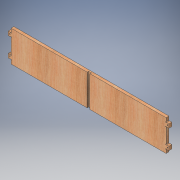
# Autodesk Inventor part: shelf
Saved by Autodesk Inventor 2016 (Build 200138000, 138)
## iProperties
Created: 2017-03-13
Part Number: shelf
Material: Wood (Birch)
Document SubType Name: Modeling
Designer: jwillauer
Density: 0.55 g/cm^3
Appearance: Birch - Natural Polished
Author: jwillauer
Autodesk Inventor part; units mm, degrees
ref_plane "YZ Plane" through (0, 0, 0) normal (1, 0, 0) x (0, 1, 0)
ref_plane "XZ Plane" through (0, 0, 0) normal (0, 1, 0) x (-1, 0, 0)
ref_plane "XY Plane" through (0, 0, 0) normal (0, 0, 1) x (1, 0, 0)
sketch "Sketch1" plane through (0, 0, 0) normal (0, 0, 1) x (1, 0, 0)
  line L0 (-759.3317, 185.2455) -> (256.6683, 185.2455)
  line L1 (-759.3317, -17.9545) -> (256.6683, -17.9545)
  line L2 (-759.3317, 185.2455) -> (-759.3317, 159.8455)
  line L3 (-759.3317, 159.8455) -> (-778.1277, 159.8455)
  line L4 (-778.1277, 159.8455) -> (-778.1277, 134.4455)
  line L5 (-778.1277, 134.4455) -> (-759.3317, 134.4455)
  line L6 (-759.3317, 134.4455) -> (-759.3317, 32.8455)
  line L7 (-759.3317, 32.8455) -> (-778.1277, 32.8455)
  line L8 (-778.1277, 32.8455) -> (-778.1277, 7.4455)
  line L9 (-778.1277, 7.4455) -> (-759.3317, 7.4455)
  line L10 (-759.3317, 7.4455) -> (-759.3317, -17.9545)
  line L11 (256.6683, 185.2455) -> (256.6683, 159.8455)
  line L12 (256.6683, 159.8455) -> (275.4643, 159.8455)
  line L13 (275.4643, 159.8455) -> (275.4643, 134.4455)
  line L14 (275.4643, 134.4455) -> (256.6683, 134.4455)
  line L15 (256.6683, 134.4455) -> (256.6683, 32.8455)
  line L16 (256.6683, 32.8455) -> (275.4643, 32.8455)
  line L17 (275.4643, 32.8455) -> (275.4643, 7.4455)
  line L18 (275.4643, 7.4455) -> (256.6683, 7.4455)
  line L19 (256.6683, 7.4455) -> (256.6683, -17.9545)
  point P0 (0, 0)
  dimension "d0" = 1016
  dimension "d1" = 203.2
  dimension "d2" = 25.4
  dimension "d3" = 25.4
  dimension "d4" = 25.4
  dimension "d5" = 25.4
  dimension "d6" = 18.796
  dimension "d7" = 18.796
  dimension "d8" = 18.796
  dimension "d9" = 25.4
  dimension "d11" = 25.4
  dimension "d12" = 25.4
  dimension "d15" = 25.4
  constraints: 40 end point, 12 perpendicular, 8 point on line, 2 parallel, 2 vertical, 1 horizontal
  measures "d0" distance of L0.start L0.end
  measures "d1" distance between parallel lines of L0 L1
  measures "d2" distance of L0.start L2.end
  measures "d3" distance of L3.end L4.end
  measures "d4" distance of L9.end L1.start
  measures "d5" distance of L7.end L8.end
  measures "d6" distance of L6.end L7.end
  measures "d7" distance of L8.end L9.end
  measures "d8" distance of L11.end L12.end
  measures "d9" distance of L0.end L11.end
  measures "d11" distance of L16.end L17.end
  measures "d12" distance of L12.end L13.end
  measures "d15" distance of L18.end L1.end
extrude "Extrusion1" add sketch "Sketch1" along normal blind 18.796
sketch "Sketch2" plane through (0, 0, 18.796) normal (0, 0, 1) x (1, 0, 0)
  line L0 (-778.1277, 159.8455) -> (-759.3317, 159.8455) projected
  line L1 (275.4643, 159.8455) -> (256.6683, 159.8455) projected
  point P0 (0, 0)
  point P1 (-759.3317, 134.5414)
  point P2 (-759.3317, 32.5902)
  point P3 (-759.3317, 7.3202)
  point P4 (256.6683, 134.5414)
  point P5 (256.6683, 32.5902)
  point P6 (256.6683, 7.3202)
hole "Hole1" at (-759.3317, 159.8455, 18.796) at (-759.3317, 134.5414, 18.796) at (-759.3317, 32.5902, 18.796) at (-759.3317, 7.3202, 18.796) at (256.6683, 159.8455, 18.796) at (256.6683, 134.5414, 18.796) at (256.6683, 32.5902, 18.796) at (256.6683, 7.3202, 18.796) direction (0, 0, -1) diameter 6.35 end through all
sketch "Sketch3" plane through (0, 0, 18.796) normal (0, 0, 1) x (1, 0, 0)
  line L0 (-778.1277, 159.8455) -> (-778.1277, 134.4455) projected
  line L1 (-778.1277, 32.8455) -> (-778.1277, 7.4455) projected
  line L2 (-762.4964, 32.8455) -> (-778.1277, 32.8455) projected
  line L3 (-778.1277, 134.4455) -> (-762.5052, 134.4455) projected
  line L4 (275.4643, 159.8455) -> (275.4643, 134.4455) projected
  line L5 (275.4643, 159.8455) -> (259.8433, 159.8455) projected
  line L6 (275.4643, 32.8455) -> (259.833, 32.8455) projected
  line L7 (275.4643, 32.8455) -> (275.4643, 7.4455) projected
  point P0 (0, 0)
  point P1 (266.0663, 147.1455)
  point P2 (266.0663, 20.1455)
  point P3 (-768.7297, 20.1455)
  point P4 (-768.7297, 147.1455)
  dimension "d25" = 9.398
  dimension "d26" = 9.398
  dimension "d27" = 12.7
  dimension "d28" = 12.7
  dimension "d29" = 9.398
  dimension "d30" = 12.7
  dimension "d31" = 12.7
  dimension "d32" = 9.398
  measures "d25" distance from line of L0 point (-768.73, 147.145)
  measures "d26" distance from line of point (-768.73, 20.145) L1
  measures "d27" distance from line of L2 point (-768.73, 20.145)
  measures "d28" distance from line of L3 point (-768.73, 147.145)
  measures "d29" distance from line of L4 point (266.066, 147.145)
  measures "d30" distance from line of L5 point (266.066, 147.145)
  measures "d31" distance from line of L6 point (266.066, 20.145)
  measures "d32" distance from line of L7 point (266.066, 20.145)
hole "Hole2" at (266.0663, 147.1455, 18.796) at (266.0663, 20.1455, 18.796) at (-768.7297, 20.1455, 18.796) at (-768.7297, 147.1455, 18.796) direction (0, 0, -1) diameter 6.35 end through all
sketch "Sketch4" plane through (0, 0, 18.796) normal (0, 0, 1) x (1, 0, 0)
  line L0 (-759.3317, 185.2455) -> (256.6683, 185.2455) projected
  line L1 (-251.3317, 185.2455) -> (-251.3317, -17.9545)
  line L2 (256.6683, -17.9545) -> (-759.3317, -17.9545) projected
  line L3 (-260.7297, 185.2455) -> (-260.7297, -17.9545)
  line L4 (-241.9337, 185.2455) -> (-241.9337, -17.9545)
  line L5 (-260.7297, 185.2455) -> (-241.9337, 185.2455)
  line L6 (-260.7297, -17.9545) -> (-241.9337, -17.9545)
  point P0 (0, 0)
  dimension "d40" = 9.398
  dimension "d41" = 9.398
  constraints: 10 end point, 3 parallel, 2 midpoint, 1 perpendicular
  measures "d40" distance between parallel lines of L1 L3
  measures "d41" distance between parallel lines of L1 L4
extrude "Extrusion2" cut sketch "Sketch4" against normal blind 9.398
body "Solid1"
